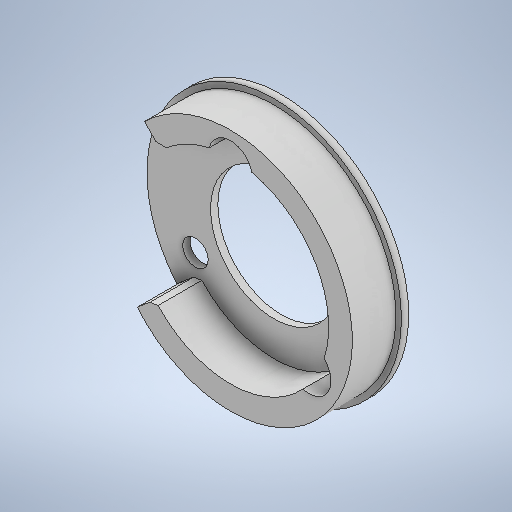
# Autodesk Inventor part: pulleycase
Saved by Autodesk Inventor 2025.2 (Build 292293000, 293)
## iProperties
Created: 2025-01-24
Part Number: pulleycase
Material: Generic
Document SubType Name: Modeling
Designer: email
Density: 1 g/cm^3
Appearance: Default
Author: email
Autodesk Inventor part; units mm, degrees
ref_plane "YZ Plane" through (0, 0, 0) normal (1, 0, 0) x (0, 1, 0)
ref_plane "XZ Plane" through (0, 0, 0) normal (0, 1, 0) x (-1, 0, 0)
ref_plane "XY Plane" through (0, 0, 0) normal (0, 0, 1) x (1, 0, 0)
sketch "Sketch1" plane through (0, 0, 0) normal (0, 0, 1) x (1, 0, 0)
  circle A0 centre (0, 25) radius 3.5
  circle A1 centre (-21.6506, -12.5) radius 3.5
  circle A2 centre (21.6506, -12.5) radius 3.5
  line L0 (0, -16) -> (0, 10.5643) construction
  circle A3 centre (0, 0) radius 17.5
  circle A4 centre (0, 0) radius 35
  arc A5 (-19.6928, -15.4012) -> (19.6928, -15.4012) centre (0, 0) ccw
  arc A6 (23.1842, -9.3538) -> (3.4914, 24.755) centre (0, 0) ccw
  arc A7 (-3.4914, 24.755) -> (-23.1842, -9.3538) centre (0, 0) ccw
  dimension "d1" = 7
  dimension "d4" = 360
  dimension "d10" = 70
  dimension "d11" = 35
  constraints: 12 point on circle, 8 centre point, 3 coincident, 2 end point, 1 vertical, 1 vertical alignment, 7 other
  measures "d1" diameter of A0
  measures "d10" diameter of A4
  measures "d11" diameter of A3
extrude "Extrusion1" add sketch "Sketch1" along normal blind 2 contours A0 A6 A2 A5 A1 A7 | A4
sketch "Sketch2" plane through (0, 0, 2) normal (0, 0, 1) x (1, 0, 0)
  circle A0 centre (0, 0) radius 27
  circle A1 centre (0, 0) radius 33.5
  line L0 (0, 0) -> (-23.6881, 23.6881)
  line L1 (0, 0) -> (-25.6625, -21.5334)
  line L2 (0, -27) -> (0, 12.4215) construction
  circle A2 centre (0, 25) radius 3.5 projected
  circle A3 centre (0, 25) radius 6
  circle A4 centre (21.6506, -12.5) radius 3.5 projected
  circle A5 centre (21.6506, -12.5) radius 6
  circle A6 centre (-21.6506, -12.5) radius 3.5 projected
  circle A7 centre (-21.6506, -12.5) radius 6
  point P0 (-20.6832, -17.3553)
  point P1 (-19.0919, 19.0919)
  point P2 (-19.9065, -18.2409)
  point P3 (-22.0329, -18.4878)
  point P4 (-5.8438, 26.36)
  point P5 (5.8438, 26.36)
  point P6 (25.7503, -8.1191)
  point P7 (19.9065, -18.2409)
  dimension "d14" = 54
  dimension "d15" = 67
  dimension "d17" = 50
  dimension "d18" = 45
  dimension "d24" = 12
  dimension "d25" = 12
  dimension "d26" = 12
  constraints: 6 end point, 5 coincident, 4 centre point, 2 point on circle, 1 point on line, 1 vertical, 3 other
  measures "d15" diameter of A1
  measures "d17" angle of L2 L1
  measures "d18" angle of L2 L0
  measures "d24" diameter of A3
  measures "d25" diameter of A5
  measures "d26" diameter of A7
extrude "Extrusion2" add sketch "Sketch2" along normal blind 12 contours A0 A3 L0 A1 L1 A7 A5
chamfer "Chamfer1" distance 2 angle 45 1 edges at (-19.0919, 19.0919, 8)
equation "\"d19\" = d24"
body "Solid1"
